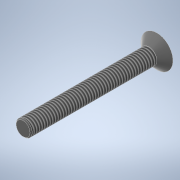
# Autodesk Inventor part: M3 x 16mm FHCS
Saved by Autodesk Inventor 2022 (Build 260153000, 153)
## iProperties
Created: 2021-10-06
Part Number: M3 x 16mm FHCS
Material: Generic
Document SubType Name: Modeling
Designer: Administrator
Density: 1 g/cm^3
Appearance: Smooth - Black
Title: DIN 912 M3 10 mm
Author: Administrator
Autodesk Inventor part; units mm, degrees
ref_plane "YZ Plane" through (0, 0, 0) normal (1, 0, 0) x (0, 1, 0)
ref_plane "XZ Plane" through (0, 0, 0) normal (0, 1, 0) x (-1, 0, 0)
ref_plane "XY Plane" through (0, 0, 0) normal (0, 0, 1) x (1, 0, 0)
sketch "Sketch1" plane through (0, 0, 0) normal (1, 0, 0) x (0, 1, 0)
  line L0 (0, 0) -> (0, -25)
  line L1 (0, -25) -> (3, -25)
  line L2 (3, -25) -> (1.5, -23.5)
  line L3 (1.5, -23.5) -> (1.5, 0)
  line L4 (1.5, 0) -> (0, 0)
  dimension "d0" = 6
  dimension "d1" = 25
  dimension "d2" = 45
  dimension "d3" = 3
  constraints: 10 end point, 2 horizontal, 1 perpendicular, 1 vertical
  measures "d0" diameter of L1.end L0
  measures "d1" distance between parallel lines of L4 L1
  measures "d2" angle of L1 L2
  measures "d3" diameter of L3 L0
revolve "Revolution1" add sketch "Sketch1" angle 360 about axis through (0, 0, 0) along (0, 0, -1)
chamfer "Chamfer1" distance 0.2 angle 45 1 edges at (0, -1.5, 0)
thread "Thread1" size "M3x0.5" class "6g" standard "ANSI Metric M Profile" full length
sketch "Sketch2" plane through (0, 0, -25) normal (0, 0, -1) x (-1, 0, 0)
  circle A0 centre (0, 0) radius 1.3 projected
  line L0 (1.1547, 0) -> (0.5774, -1)
  line L1 (0.5774, -1) -> (-0.5774, -1)
  line L2 (-0.5774, -1) -> (-1.1547, 0)
  line L3 (-1.1547, 0) -> (-0.5774, 1)
  line L4 (-0.5774, 1) -> (0.5774, 1)
  line L5 (0.5774, 1) -> (1.1547, 0)
  dimension "d10" = 2
  constraints: 12 end point, 1 coincident, 1 horizontal, 13 other
  measures "d10" distance between parallel lines of L1 L4
extrude "Extrusion1" cut sketch "Sketch2" against normal blind 1.2 contours L0 L1 L2 L3 L4 L5
body "Solid2"
